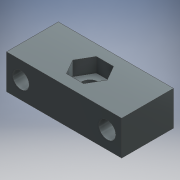
# Autodesk Inventor part: back_sprocket_holder
Saved by Autodesk Inventor 2016 (Build 200138000, 138)
## iProperties
Created: 2017-01-06
Part Number: back_sprocket_holder
Material: Generic
Document SubType Name: Modeling
Designer: hesaon
Density: 1 g/cm^3
Appearance: Default
Author: hesaon
Autodesk Inventor part; units mm, degrees
ref_plane "YZ Plane" through (0, 0, 0) normal (1, 0, 0) x (0, 1, 0)
ref_plane "XZ Plane" through (0, 0, 0) normal (0, 1, 0) x (-1, 0, 0)
ref_plane "XY Plane" through (0, 0, 0) normal (0, 0, 1) x (1, 0, 0)
sketch "Sketch1" plane through (0, 0, 0) normal (0, 1, 0) x (-1, 0, 0)
  line L0 (0, 0) -> (40, 0)
  line L1 (40, 0) -> (40, -12)
  line L2 (40, -12) -> (0, -12)
  line L3 (0, -12) -> (0, 0)
  circle A0 centre (35, -6) radius 2.85
  circle A1 centre (5, -6) radius 2.95
  dimension "d0" = 40
  dimension "d1" = 12
  dimension "d2" = 5.7
  dimension "d3" = 5.9
  dimension "d4" = 5
  dimension "d6" = 6
  dimension "d33" = 5
  constraints: 8 end point, 2 centre point, 2 parallel, 1 horizontal, 1 horizontal alignment, 1 perpendicular
  measures "d0" distance of L1.end L2.end
  measures "d1" distance of L0.end L1.end
  measures "d2" diameter of A0
  measures "d3" diameter of A1
  measures "d4" distance from line of L1 A0.centre
  measures "d6" distance from line of L2 A0.centre
  measures "d33" distance from line of L3 A1.centre
extrude "Extrusion1" add sketch "Sketch1" along normal blind 18
sketch "Sketch8" plane through (-40, 0, 0) normal (0, 0, 1) x (1, 0, 0)
  circle A0 centre (20, 9) radius 2.95
  line L0 (0, 0) -> (0, 18) projected
  line L1 (40, 0) -> (0, 0) projected
  dimension "d34" = 5.9
  dimension "d35" = 20
  dimension "d36" = 9
  constraints: 1 centre point
  measures "d34" diameter of A0
  measures "d35" distance from line of L0 A0.centre
  measures "d36" distance from line of L1 A0.centre
extrude "Extrusion8" cut sketch "Sketch8" against normal up to next
sketch "Sketch9" plane through (-40, 0, 0) normal (0, 0, 1) x (1, 0, 0)
  circle A0 centre (20, 9) radius 2.95 projected
  line L0 (16.9978, 3.8) -> (13.9956, 9)
  line L1 (13.9956, 9) -> (16.9978, 14.2)
  line L2 (16.9978, 14.2) -> (23.0022, 14.2)
  line L3 (23.0022, 14.2) -> (26.0044, 9)
  line L4 (26.0044, 9) -> (23.0022, 3.8)
  line L5 (23.0022, 3.8) -> (16.9978, 3.8)
  line L6 (40, 0) -> (0, 0) projected
  dimension "d39" = 10.4
  constraints: 12 end point, 1 coincident, 1 parallel, 13 other
  measures "d39" distance between parallel lines of L0 L3
extrude "Extrusion9" cut sketch "Sketch9" against normal blind 5
body "Solid1"
